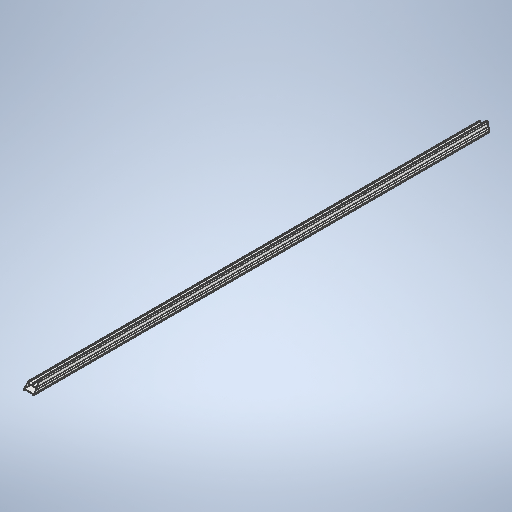
# Autodesk Inventor part: SP40-01 MARCO BATIENTE - PAÑO FIJO 2100MM
Saved by Autodesk Inventor 2025 (Build 290162000, 162)
## iProperties
Created: 2026-01-17
Part Number: SP40-01 MARCO BATIENTE - PAÑO FIJO 2100MM
Material: Aluminio
Document SubType Name: Modeling
Designer: ROLANDO
Density: 2.7 g/cm^3
Appearance: Satinado
Author: ROLANDO
Autodesk Inventor part; units mm, degrees
ref_plane "YZ Plane" through (0, 0, 0) normal (1, 0, 0) x (0, 1, 0)
ref_plane "XZ Plane" through (0, 0, 0) normal (0, 1, 0) x (-1, 0, 0)
ref_plane "XY Plane" through (0, 0, 0) normal (0, 0, 1) x (1, 0, 0)
sketch "Boceto1" plane through (0, 0, 0) normal (0, 0, 1) x (1, 0, 0)
  line L0 (-45, 21.0335) -> (-45, 0)
  line L1 (-43.1, 4) -> (-1.9, 4)
  line L2 (0, 0) -> (0, 15.6335)
  line L3 (-4.7, 44) -> (-4.7, 21.4102)
  line L4 (-4.7, 44) -> (-9.9, 44)
  line L5 (-8.5, 42.6) -> (-6.1, 42.6)
  line L6 (-6.1, 36.1) -> (-8.5, 36.1)
  line L7 (-43.6, 19.6335) -> (-5.4, 19.6335)
  line L8 (-1.4, 15.6335) -> (-1.4, 5.9)
  line L9 (-1.9, 5.4) -> (-43.1, 5.4)
  line L10 (-43.6, 5.9) -> (-43.6, 19.6335)
  arc A0 (0, 15.6335) -> (-4.3017, 20.9206) centre (-5.4, 15.6335) ccw
  arc A1 (-1.4, 15.6335) -> (-5.4, 19.6335) centre (-5.4, 15.6335) ccw
  line L11 (-1.4, 3.5) -> (-1.4, 1.7468)
  line L12 (-2.5, 0) -> (0, 0)
  line L13 (-6.1, 21.5) -> (-6.1, 34.7)
  line L14 (-6.1, 36.1) -> (-6.1, 42.6)
  line L15 (-43.6, 3.5) -> (-43.6, 1.6777)
  line L16 (-42.5, 0) -> (-45, 0)
  line L17 (-42.5, 0) -> (-42.5, 0.4554)
  line L18 (-2.5, 0) -> (-2.5, 0.7)
  line L19 (-43.6, 21) -> (-43.6, 24)
  line L20 (-42.48, 25.4) -> (-45, 25.4)
  line L21 (-45, 25.4) -> (-45, 21.0335)
  line L22 (-24, 21) -> (-24, 25.4)
  line L23 (-24, 25.4) -> (-26.39, 25.4)
  line L24 (-25.4, 24) -> (-25.4, 21)
  line L25 (-6.6, 21) -> (-24, 21)
  line L26 (-25.4, 21) -> (-43.6, 21)
  line L27 (-41.6, 24) -> (-43.6, 24)
  line L28 (-27.4, 24) -> (-25.4, 24)
  line L29 (-42.7447, 0.8853) -> (-43.3553, 1.2478)
  line L30 (-2.5, 0.7) -> (-1.6082, 1.3408)
  line L31 (-41.6, 24) -> (-41.6, 24.695)
  line L32 (-27.4, 24) -> (-27.4, 24.7058)
  line L33 (-42.48, 25.4) -> (-41.6, 24.695)
  line L34 (-27.4, 24.7058) -> (-26.39, 25.4)
  line L35 (-6.1, 34.7) -> (-9.9, 34.7)
  line L36 (-8.5, 37.35) -> (-8.5, 36.1)
  line L37 (-8.5, 41.35) -> (-8.5, 42.6)
  line L38 (-8.5, 37.35) -> (-9.2058, 37.35)
  line L39 (-8.5, 41.35) -> (-9.2058, 41.35)
  line L40 (-9.9, 44) -> (-9.9, 42.36)
  line L41 (-9.9, 42.36) -> (-9.2058, 41.35)
  line L42 (-9.9, 34.7) -> (-9.9, 36.34)
  line L43 (-9.9, 36.34) -> (-9.2058, 37.35)
  arc A2 (-6.6, 21) -> (-6.1, 21.5) centre (-6.6, 21.5) ccw
  arc A3 (-4.7, 21.4102) -> (-4.3017, 20.9206) centre (-4.2, 21.4102) ccw
  arc A4 (-1.9, 5.4) -> (-1.4, 5.9) centre (-1.9, 5.9) ccw
  arc A5 (-1.4, 3.5) -> (-1.9, 4) centre (-1.9, 3.5) ccw
  arc A6 (-1.6082, 1.3408) -> (-1.4, 1.7468) centre (-1.9, 1.7468) ccw
  arc A7 (-43.6, 5.9) -> (-43.1, 5.4) centre (-43.1, 5.9) ccw
  arc A8 (-43.1, 4) -> (-43.6, 3.5) centre (-43.1, 3.5) ccw
  arc A9 (-43.6, 1.6777) -> (-43.3553, 1.2478) centre (-43.1, 1.6777) ccw
  line L44 (0, 4) -> (0, 4.0335)
  arc A10 (-42.5, 0.4554) -> (-42.7447, 0.8853) centre (-43, 0.4554) ccw
  point P0 (-8.5, 41.975)
  point P1 (-42.5, 4)
  point P2 (-6.1, 39.35)
  point P3 (-42.5, 0.74)
  dimension "d16" = 5.4
  dimension "d17" = 4
  dimension "d32" = 1.4
  dimension "d35" = 1.4
  dimension "d37" = 3
  dimension "d38" = 25.4
  dimension "d44" = 18.2
  dimension "d50" = 0.7
  dimension "d53" = 40.3
  dimension "d54" = 37.5
  dimension "d55" = 1.4
  dimension "d57" = 17
  dimension "d62" = 30.7
  dimension "d63" = 35.7
  dimension "d64" = 4.4
  dimension "d66" = 3
  dimension "d69" = 4.4
  dimension "d71" = 3.4
  dimension "d72" = 3.4
  dimension "d73" = 0.88
  dimension "d74" = 1.01
  dimension "d75" = 34.5
  dimension "d76" = 38.7
  dimension "d77" = 0.695
  dimension "d78" = 0.7058
  dimension "d81" = 23
  dimension "d82" = 44
  dimension "d84" = 6.5
  dimension "d85" = 2.4
  dimension "d86" = 2.4
  dimension "d87" = 9.3
  dimension "d88" = 1.4
  dimension "d99" = 1.4
  dimension "d100" = 1.4
  dimension "d102" = 1.4
  dimension "d140" = 111
  dimension "d141" = 4
  dimension "d142" = 6.02
  dimension "d143" = 0.7058
  dimension "d144" = 0.7058
  dimension "d199" = 1.4
  dimension "d201" = 14.2
  dimension "d202" = 0.5
  dimension "d203" = 3.01
  dimension "d204" = 2
  dimension "d205" = 2.5
  dimension "d206" = 4.7
  dimension "d207" = 6.1
  dimension "d208" = 42.5
  dimension "d209" = 41.35
  dimension "d210" = 5.4
  dimension "d211" = 4
  dimension "d212" = 19.6335
  dimension "d216" = 4.0335
  dimension "d218" = 0.74
  dimension "d219" = 0.5
  dimension "d220" = 45
  dimension "d221" = 5.2
  constraints: 90 end point, 22 point on circle, 21 tangent, 13 parallel, 11 centre point, 9 horizontal, 7 equal radius, 6 perpendicular, 5 collinear, 5 point on line, 4 vertical, 2 coincident, 2 midpoint, 1 equal length
  measures "d16" radius of A0
  measures "d17" radius of A1
  measures "d32" distance between parallel lines of L22 L24
  measures "d35" distance between parallel lines of L19 L21
  measures "d37" distance between parallel lines of L26 L28
  measures "d38" distance between parallel lines of L16 L20
  measures "d44" distance between parallel lines of L24 L19
  measures "d50" distance of L12.start L18.end
  measures "d53" distance between parallel lines of L0 L3
  measures "d54" distance between parallel lines of L10 L14
  measures "d55" distance between parallel lines of L3 L14
  measures "d57" distance between parallel lines of L1 L26
  measures "d62" angle of L16 L29
  measures "d63" angle of L12 L30
  measures "d64" distance between parallel lines of L20 L26
  measures "d66" distance between parallel lines of L26 L27
  measures "d69" distance between parallel lines of L26 L23
  measures "d71" distance between parallel lines of L22 L32
  measures "d72" distance between parallel lines of L21 L31
  measures "d73" distance from line of L31 L20.start
  measures "d74" distance from line of L32 L23.end
  measures "d75" angle of L23 L34
  measures "d76" angle of L20 L33
  measures "d77" distance of L27.start L31.end
  measures "d78" distance of L28.start L32.end
  measures "d81" distance between parallel lines of L25 L4
  measures "d82" distance between parallel lines of L12 L4
  measures "d84" distance between parallel lines of L6 L5
  measures "d85" distance from line of L5.start L14
  measures "d86" distance of L6.start L6.end
  measures "d87" distance between parallel lines of L35 L4
  measures "d88" distance between parallel lines of L35 L6
  measures "d99" distance between parallel lines of L4 L5
  measures "d100" distance from line of point (-8.5, 41.975) L40
  measures "d102" distance between parallel lines of L36 L42
  measures "d140" angle of L43 L41
  measures "d141" distance between parallel lines of L38 L39
  measures "d142" distance of L42.end L40.end
  measures "d143" distance of L37.start L39.end
  measures "d144" distance of L36.start L38.end
  measures "d199" radial gap between concentric circles of A0 A1
  measures "d201" distance between parallel lines of L32 L31
  measures "d202" radius of A2
  measures "d203" vertical distance of point (-6.1, 39.35) L40.end
  measures "d204" distance from line of point (-6.1, 39.35) L39
  measures "d205" distance between parallel lines of L2 L18
  measures "d206" distance between parallel lines of L2 L3
  measures "d207" distance between parallel lines of L2 L14
  measures "d208" distance between parallel lines of L2 L17
  measures "d209" distance between parallel lines of L12 L39
  measures "d210" distance between parallel lines of L9 L12
  measures "d211" distance between parallel lines of L1 L12
  measures "d212" distance between parallel lines of L7 L12
  measures "d216" distance from line of L44.end L12
  measures "d218" distance of L16.start point (-42.5, 0.74)
  measures "d219" radius of A10
  measures "d220" distance between parallel lines of L2 L0
  measures "d221" distance between parallel lines of L40 L3
extrude "Extrusión1" add sketch "Boceto1" against normal blind 2100
sketch "Boceto2" plane through (0, 0, 0) normal (1, 0, 0) x (0, 1, 0)
  line L0 (0, 0) -> (15.6335, 0) projected
  line L1 (0, 0) -> (0, -2100) projected
  line L2 (15.6335, -2100) -> (0, -2100) projected
  line L3 (15.6335, 0) -> (15.6335, -2100) projected
  line L4 (15.6335, 0) -> (20.9206, 0) projected
  line L5 (15.6335, 0) -> (15.6335, -2100) projected
  line L6 (20.9206, -2100) -> (15.6335, -2100) projected
  line L7 (20.9206, 0) -> (20.9206, -2100) projected
  line L8 (20.9206, 0) -> (21.4102, 0) projected
  line L9 (20.9206, 0) -> (20.9206, -2100) projected
  line L10 (21.4102, -2100) -> (20.9206, -2100) projected
  line L11 (21.4102, 0) -> (21.4102, -2100) projected
  line L12 (21.4102, 0) -> (44, 0) projected
  line L13 (21.4102, 0) -> (21.4102, -2100) projected
  line L14 (44, -2100) -> (21.4102, -2100) projected
  line L15 (44, 0) -> (44, -2100) projected
  line L16 (0, 0) -> (44, -44)
  line L17 (44, 0) -> (44, -44)
  line L18 (0, 0) -> (44, 0)
  dimension "d222" = 45
  constraints: 6 end point, 2 collinear, 1 point on line
  measures "d222" angle of L16 L18
extrude "Extrusión2" cut sketch "Boceto2" against normal through all contours L0 L3 L16 | L4 L7 L16 L3 | L8 L11 L16 L7 | L12 L15 L16 L11
